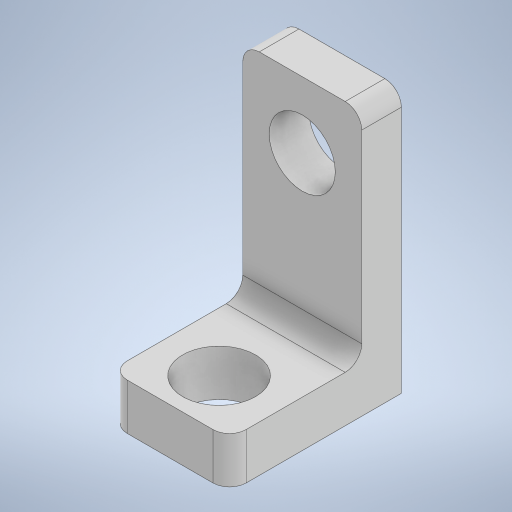
# Autodesk Inventor part: driver-bracket
Saved by Autodesk Inventor 2024 (Build 280153000, 153)
## iProperties
Created: 2024-05-12
Part Number: driver-bracket
Material: Generic
Document SubType Name: Modeling
Designer: MaartenGeorgesBuelen
Density: 1 g/cm^3
Appearance: Default
Author: MaartenGeorgesBuelen
## iProperties of the stored document driver-bracket_3DPrint.ipt
Created: 2024-05-12
Part Number: driver-bracket_3DPrint
Material: Generic
Document SubType Name: Modeling
Designer: MaartenGeorgesBuelen
Density: 1 g/cm^3
Appearance: Default
Author: MaartenGeorgesBuelen
Autodesk Inventor part; units mm, degrees
ref_plane "YZ Plane" through (0, 0, 0) normal (1, 0, 0) x (0, 1, 0)
ref_plane "XZ Plane" through (0, 0, 0) normal (0, 1, 0) x (-1, 0, 0)
ref_plane "XY Plane" through (0, 0, 0) normal (0, 0, 1) x (1, 0, 0)
sketch "Sketch1" plane through (0, 0, 0) normal (0, 0, 1) x (1, 0, 0)
  circle A0 centre (0, 0) radius 2.5
  line L0 (-4.5, 5) -> (4.5, 5)
  line L1 (4.5, 5) -> (4.5, -11.5)
  line L2 (4.5, -11.5) -> (-4.5, -11.5)
  line L3 (-4.5, -11.5) -> (-4.5, 5)
  line L4 (-4.5, -11.5) -> (4.5, -11.5)
  line L5 (4.5, -11.5) -> (4.5, -15)
  line L6 (4.5, -15) -> (-4.5, -15)
  line L7 (-4.5, -15) -> (-4.5, -11.5)
  dimension "d0" = 5
  dimension "d1" = 4.5
  dimension "d2" = 4.5
  dimension "d3" = 5
  dimension "d4" = 11.5
  dimension "d5" = 3.5
  constraints: 16 end point, 4 parallel, 2 horizontal, 2 perpendicular, 1 centre point, 1 coincident
  measures "d0" diameter of A0
  measures "d1" distance from line of point (0, 0) L3
  measures "d2" distance from line of L1 point (0, 0)
  measures "d3" distance from line of point (0, 0) L0
  measures "d4" distance from line of L2 point (0, 0)
  measures "d5" distance of L4.end L5.end
extrude "Extrusion1" add sketch "Sketch1" along normal blind 3
sketch "Sketch2" plane through (0, 0, 3) normal (0, 0, 1) x (1, 0, 0)
  line L0 (4.5, 5) -> (-4.5, 5) projected
  line L1 (-4.5, 5) -> (-4.5, -15) projected
  line L2 (-4.5, -15) -> (4.5, -15) projected
  line L3 (4.5, -15) -> (4.5, 5) projected
  circle A0 centre (0, 0) radius 2.5 projected
  line L4 (-4.5, -15) -> (4.5, -15)
  line L5 (4.5, -15) -> (4.5, -11.5)
  line L6 (4.5, -11.5) -> (-4.5, -11.5)
  line L7 (-4.5, -11.5) -> (-4.5, -15)
  dimension "d8" = 3.5
  constraints: 8 end point, 2 parallel, 1 horizontal, 1 perpendicular, 1 point on line
  measures "d8" distance of L5.end L4.end
extrude "Extrusion2" add sketch "Sketch2" along normal blind 10 contours L3 L2 L1 L6
sketch "Sketch3" plane through (-4.5, -11.5, 3) normal (0, 1, 0) x (1, 0, 0)
  point P0 (4.5, 3)
  point P1 (4.4515, -6.2435)
hole "Hole1" at (-0.0485, -11.5, 9.2435) direction (0, -1, 0) diameter 5.5 depth 4 tip angle 118
fillet "Fillet1" radius 1.25 5 edges at (4.5, -13.25, 13) (-4.5, -13.25, 13) (0, -11.5, 3) (4.5, 5, 1.5) (-4.5, 5, 1.5)
body "Solid1"
